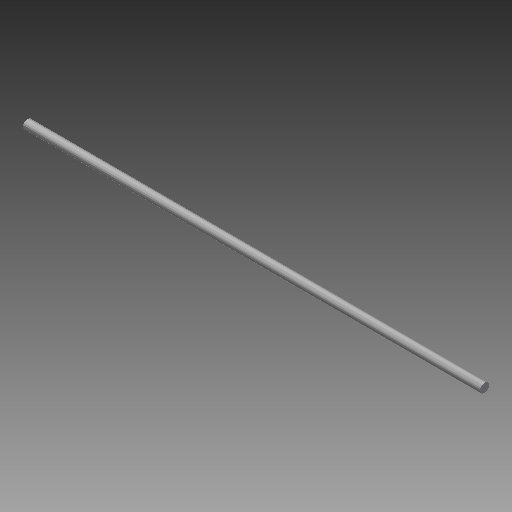
# Autodesk Inventor part: Shaft
Saved by Autodesk Inventor 2019.4 (Build 234330000, 330)
## iProperties
Created: 2020-01-09
Part Number: Shaft
Material: Steel
Document SubType Name: Modeling
Designer: Mark
Mass: 2466.15 g
Surface Area: 634.602 cm^2
Volume: 314.159 cm^3
Density: 7.85 g/cm^3
Appearance: Steel
CustomPartVersion: 1
Author: Mark
Length: 1000.000 mm
Autodesk Inventor part; units mm, degrees
ref_plane "Start Plane" through (0, 0, 0) normal (1, 0, 0) x (0, 1, 0)
ref_plane "XZ Plane" through (0, 0, 0) normal (0, 1, 0) x (-1, 0, 0)
ref_plane "XY Plane" through (0, 0, 0) normal (0, 0, 1) x (1, 0, 0)
sketch "Main Sketch" plane through (0, 0, 0) normal (0, 0, 1) x (1, 0, 0)
  line L0 (0, 0) -> (1000, 0)
  line L1 (0, 0) -> (0, 10)
  line L2 (1000, 10) -> (1000, 0)
  line L3 (0, 10) -> (1000, 10)
  dimension "d3" = 20
  constraints: 8 end point, 2 horizontal, 2 vertical
  measures "d3" diameter of L3 L0
revolve "Revolution1" add sketch "Main Sketch" angle 360 about axis through (0, 0, 0) along (1, 0, 0)
equation "\"Length\" = 1000"
body "Solid1"
